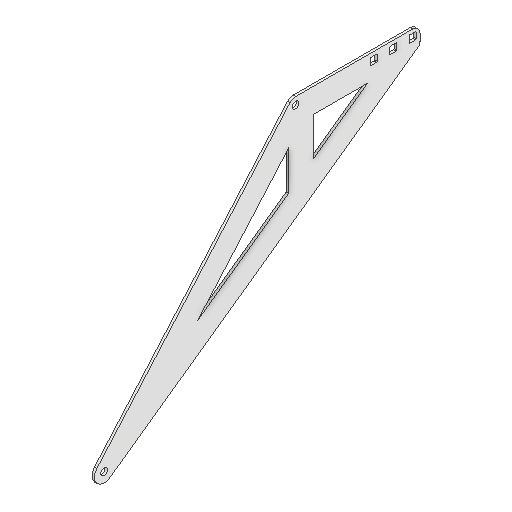
# Autodesk Inventor part: Triiangle Gusset
Saved by Autodesk Inventor 2025 (Build 290162000, 162)
## iProperties
Created: 2025-02-15
Part Number: Triiangle Gusset
Material: Acetal Resin, White
Document SubType Name: Modeling
Designer: Averey Ku
Density: 1.425 g/cm^3
Appearance: Smooth - White
Mass: 19.6613 g
Surface Area: 183.833 cm^2
Volume: 13.7974 cm^3
Author: Averey Ku
Autodesk Inventor part; units mm, degrees
ref_plane "YZ Plane" through (0, 0, 0) normal (1, 0, 0) x (0, 1, 0)
ref_plane "XZ Plane" through (0, 0, 0) normal (0, 1, 0) x (-1, 0, 0)
ref_plane "XY Plane" through (0, 0, 0) normal (0, 0, 1) x (1, 0, 0)
sketch "main" plane through (0, 0, 0) normal (0, 0, 1) x (1, 0, 0)
  circle A0 centre (2982.9462, -106.4126) radius 2.1844
  circle A1 centre (2838.6663, 17.9802) radius 2.1844
  arc A2 (2982.9462, -187.3751) -> (2987.7082, -182.5494) centre (2982.9462, -182.6126) ccw
  arc A3 (2987.7082, -106.4758) -> (2986.0859, -102.8316) centre (2982.9462, -106.4126) ccw
  arc A4 (2842.8526, 22.7548) -> (2833.5352, 14.2393) centre (2838.6663, 17.9802) ccw
  line L0 (2987.7082, -106.4758) -> (2987.7082, -182.5494)
  line L1 (2986.0859, -102.8316) -> (2842.8526, 22.7548)
  line L2 (2981.1428, -180.3012) -> (2984.7496, -180.3012)
  line L3 (2985.2576, -180.8092) -> (2985.2576, -184.416)
  line L4 (2984.7496, -184.924) -> (2981.1428, -184.924)
  line L5 (2980.6348, -184.416) -> (2980.6348, -180.8092)
  line L6 (2980.6348, -180.3012) -> (2985.2576, -184.924) construction
  line L7 (2985.2576, -180.3012) -> (2980.6348, -184.924) construction
  line L8 (2981.1428, -167.6012) -> (2984.7496, -167.6012)
  line L9 (2985.2576, -168.1092) -> (2985.2576, -171.716)
  line L10 (2984.7496, -172.224) -> (2981.1428, -172.224)
  line L11 (2980.6348, -171.716) -> (2980.6348, -168.1092)
  line L12 (2980.6348, -167.6012) -> (2985.2576, -172.224) construction
  line L13 (2985.2576, -167.6012) -> (2980.6348, -172.224) construction
  line L14 (2981.1428, -154.9012) -> (2984.7496, -154.9012)
  line L15 (2985.2576, -155.4092) -> (2985.2576, -159.016)
  line L16 (2984.7496, -159.524) -> (2981.1428, -159.524)
  line L17 (2980.6348, -159.016) -> (2980.6348, -155.4092)
  line L18 (2980.6348, -154.9012) -> (2985.2576, -159.524) construction
  line L19 (2985.2576, -154.9012) -> (2980.6348, -159.524) construction
  arc A5 (2984.7496, -184.924) -> (2985.2576, -184.416) centre (2984.7496, -184.416) ccw
  arc A6 (2980.6348, -184.416) -> (2981.1428, -184.924) centre (2981.1428, -184.416) ccw
  arc A7 (2981.1428, -180.3012) -> (2980.6348, -180.8092) centre (2981.1428, -180.8092) ccw
  arc A8 (2985.2576, -180.8092) -> (2984.7496, -180.3012) centre (2984.7496, -180.8092) ccw
  arc A9 (2984.7496, -172.224) -> (2985.2576, -171.716) centre (2984.7496, -171.716) ccw
  arc A10 (2980.6348, -171.716) -> (2981.1428, -172.224) centre (2981.1428, -171.716) ccw
  arc A11 (2981.1428, -167.6012) -> (2980.6348, -168.1092) centre (2981.1428, -168.1092) ccw
  arc A12 (2985.2576, -168.1092) -> (2984.7496, -167.6012) centre (2984.7496, -168.1092) ccw
  arc A13 (2984.7496, -159.524) -> (2985.2576, -159.016) centre (2984.7496, -159.016) ccw
  arc A14 (2980.6348, -159.016) -> (2981.1428, -159.524) centre (2981.1428, -159.016) ccw
  arc A15 (2981.1428, -154.9012) -> (2980.6348, -155.4092) centre (2981.1428, -155.4092) ccw
  arc A16 (2985.2576, -155.4092) -> (2984.7496, -154.9012) centre (2984.7496, -155.4092) ccw
  line L20 (2982.9462, -187.3751) -> (2978.2364, -187.3751)
  line L21 (2975.647, -186.0374) -> (2833.5352, 14.2393)
  arc A17 (2975.647, -186.0374) -> (2978.2364, -187.3751) centre (2978.2364, -184.2001) ccw
  line L22 (2961.0316, -101.9771) -> (2893.3678, -42.6497)
  line L23 (2971.8332, -117.8521) -> (2971.8332, -153.2302)
  line L24 (2961.0316, -101.9771) -> (2935.4651, -101.9771)
  line L25 (2971.8332, -117.8521) -> (2946.7297, -117.8521)
  line L26 (2893.3678, -42.6497) -> (2935.4651, -101.9771)
  line L27 (2946.7297, -117.8521) -> (2971.8332, -153.2302)
  point P0 (2935.9211, -90.1281)
  point P1 (2982.9462, -169.9126)
  point P2 (2982.9462, -157.2126)
  point P3 (2976.5962, -187.3751)
  point P4 (2959.2815, -117.8521)
  dimension "d0" = 12.7
  dimension "d1" = 9.525
  dimension "d2" = 9.525
  dimension "d7" = 4.6228
  dimension "d8" = 4.6228
  dimension "d9" = 4.6228
  dimension "d10" = 4.6228
  dimension "d11" = 4.6228
  dimension "d12" = 4.6228
  dimension "d13" = 0.508
  dimension "d14" = 6.35
  dimension "d15" = 3.175
  dimension "d18" = 15.875
  dimension "d19" = 15.875
  dimension "d20" = 15.875
  dimension "d21" = 15.875
  dimension "d22" = 15.875
  measures "d0" diameter of A4
  measures "d1" diameter of A3
  measures "d2" diameter of A2
  measures "d7" distance of L6.end L7.end
  measures "d8" distance of L7.start L6.end
  measures "d9" distance of L12.end L13.end
  measures "d10" distance of L13.start L12.end
  measures "d11" distance of L18.end L19.end
  measures "d12" distance of L19.start L18.end
  measures "d13" radius of A5
  measures "d14" distance of L20.start point (2976.596, -187.375)
  measures "d15" radius of A17
  measures "d18" distance between parallel lines of L0 L23
  measures "d19" distance between parallel lines of L22 L1
  measures "d20" distance from line of point (2959.281, -117.852) L24
  measures "d21" distance between parallel lines of L21 L26
  measures "d22" distance between parallel lines of L21 L27
sketch "Sketch1" plane through (0, 0, 0) normal (1, 0, 0) x (0, 1, 0)
  circle A0 centre (0, 76.2) radius 2.1844
  circle A1 centre (-144.2799, 200.5928) radius 2.1844
  arc A2 (0, -4.7625) -> (4.7621, 0.0632) centre (0, 0) ccw
  arc A3 (4.7621, 76.1368) -> (3.1398, 79.781) centre (0, 76.2) ccw
  arc A4 (-140.0936, 205.3674) -> (-149.411, 196.8519) centre (-144.2799, 200.5928) ccw
  line L0 (4.7621, 76.1368) -> (4.7621, 0.0632)
  line L1 (3.1398, 79.781) -> (-140.0936, 205.3674)
  line L2 (-1.8034, 2.3114) -> (1.8034, 2.3114)
  line L3 (2.3114, 1.8034) -> (2.3114, -1.8034)
  line L4 (1.8034, -2.3114) -> (-1.8034, -2.3114)
  line L5 (-2.3114, -1.8034) -> (-2.3114, 1.8034)
  line L6 (-2.3114, 2.3114) -> (2.3114, -2.3114) construction
  line L7 (2.3114, 2.3114) -> (-2.3114, -2.3114) construction
  line L8 (-1.8034, 15.0114) -> (1.8034, 15.0114)
  line L9 (2.3114, 14.5034) -> (2.3114, 10.8966)
  line L10 (1.8034, 10.3886) -> (-1.8034, 10.3886)
  line L11 (-2.3114, 10.8966) -> (-2.3114, 14.5034)
  line L12 (-2.3114, 15.0114) -> (2.3114, 10.3886) construction
  line L13 (2.3114, 15.0114) -> (-2.3114, 10.3886) construction
  line L14 (-1.8034, 27.7114) -> (1.8034, 27.7114)
  line L15 (2.3114, 27.2034) -> (2.3114, 23.5966)
  line L16 (1.8034, 23.0886) -> (-1.8034, 23.0886)
  line L17 (-2.3114, 23.5966) -> (-2.3114, 27.2034)
  line L18 (-2.3114, 27.7114) -> (2.3114, 23.0886) construction
  line L19 (2.3114, 27.7114) -> (-2.3114, 23.0886) construction
  arc A5 (1.8034, -2.3114) -> (2.3114, -1.8034) centre (1.8034, -1.8034) ccw
  arc A6 (-2.3114, -1.8034) -> (-1.8034, -2.3114) centre (-1.8034, -1.8034) ccw
  arc A7 (-1.8034, 2.3114) -> (-2.3114, 1.8034) centre (-1.8034, 1.8034) ccw
  arc A8 (2.3114, 1.8034) -> (1.8034, 2.3114) centre (1.8034, 1.8034) ccw
  arc A9 (1.8034, 10.3886) -> (2.3114, 10.8966) centre (1.8034, 10.8966) ccw
  arc A10 (-2.3114, 10.8966) -> (-1.8034, 10.3886) centre (-1.8034, 10.8966) ccw
  arc A11 (-1.8034, 15.0114) -> (-2.3114, 14.5034) centre (-1.8034, 14.5034) ccw
  arc A12 (2.3114, 14.5034) -> (1.8034, 15.0114) centre (1.8034, 14.5034) ccw
  arc A13 (1.8034, 23.0886) -> (2.3114, 23.5966) centre (1.8034, 23.5966) ccw
  arc A14 (-2.3114, 23.5966) -> (-1.8034, 23.0886) centre (-1.8034, 23.5966) ccw
  arc A15 (-1.8034, 27.7114) -> (-2.3114, 27.2034) centre (-1.8034, 27.2034) ccw
  arc A16 (2.3114, 27.2034) -> (1.8034, 27.7114) centre (1.8034, 27.2034) ccw
  line L20 (0, -4.7625) -> (-4.7098, -4.7625)
  line L21 (-7.2992, -3.4248) -> (-149.411, 196.8519)
  arc A17 (-7.2992, -3.4248) -> (-4.7098, -4.7625) centre (-4.7098, -1.5875) ccw
  line L22 (-21.9146, 80.6355) -> (-89.5784, 139.9629)
  line L23 (-11.1129, 64.7605) -> (-11.1129, 29.3823)
  line L24 (-21.9146, 80.6355) -> (-47.481, 80.6355)
  line L25 (-11.1129, 64.7605) -> (-36.2165, 64.7605)
  line L26 (-89.5784, 139.9629) -> (-47.481, 80.6355)
  line L27 (-36.2165, 64.7605) -> (-11.1129, 29.3823)
  constraints: 1 other
extrude "Extrusion1" add sketch "Sketch1" along normal blind 1.5875
body "Solid1"
